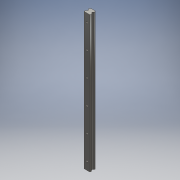
# Autodesk Inventor part: [Z] HGR15R
Saved by Autodesk Inventor 2016 (Build 200138000, 138)
## iProperties
Created: 2013-03-18
Part Number: [Z] HGR15R
Material: Сталь
Description: SolidWorks IGES file using analytic representation for surfaces
Document SubType Name: Modeling
Designer: stan
Density: 7.85 g/cm^3
Appearance: Сталь — полированная
Sending System: SolidWorks 2012
Preprocessor: SolidWorks 2012
Minimum Resolution: 0.0
Sending System Product ID: HGR15R.SLDPRT
Receiving System Product ID: HGR15R.SLDPRT
Sent Units: Millimeter
Translation Standard: IGES 5.3
Model Creation Time: 2013-03-18
Autodesk Inventor part; units mm, degrees
ref_plane "YZ Plane" through (0, 0, 0) normal (1, 0, 0) x (0, 1, 0)
ref_plane "XZ Plane" through (0, 0, 0) normal (0, 1, 0) x (-1, 0, 0)
ref_plane "XY Plane" through (0, 0, 0) normal (0, 0, 1) x (1, 0, 0)
ref_plane "РабПлоскость1" through (-6.8, -15, 75) normal (0, 0, 1) x (1, 0, 0)
sketch "Эскиз2" plane through (-6.8, -15, 75) normal (0, 0, 1) x (1, 0, 0)
  arc A0 (11.9032, 8.6142) -> (12.017, 8.8451) centre (11.6204, 8.897) ccw projected
  arc A1 (13.5419, 10.2529) -> (12.017, 8.8451) centre (13.6233, 8.6349) ccw projected
  line L0 (14.3, 11.011) -> (13.5419, 10.2529) projected
  line L1 (14.3, 12.549) -> (14.3, 11.011) projected
  line L2 (13.5304, 13.3186) -> (14.3, 12.549) projected
  arc A2 (12.0183, 14.7157) -> (13.5304, 13.3186) centre (13.6233, 14.936) ccw projected
  arc A3 (12.0183, 14.7157) -> (11.9049, 14.9441) centre (11.622, 14.6613) ccw projected
  line L3 (11.849, 15) -> (11.9049, 14.9441) projected
  line L4 (11.849, 15) -> (1.751, 15) projected
  line L5 (1.6951, 14.9441) -> (1.751, 15) projected
  arc A4 (1.6951, 14.9441) -> (1.5817, 14.7157) centre (1.978, 14.6613) ccw projected
  arc A5 (0.0696, 13.3186) -> (1.5817, 14.7157) centre (-0.0233, 14.936) ccw projected
  line L6 (-0.7, 12.549) -> (0.0696, 13.3186) projected
  line L7 (-0.7, 11.011) -> (-0.7, 12.549) projected
  line L8 (0.0581, 10.2529) -> (-0.7, 11.011) projected
  arc A6 (1.583, 8.8451) -> (0.0581, 10.2529) centre (-0.0233, 8.6349) ccw projected
  arc A7 (1.583, 8.8451) -> (1.6968, 8.6142) centre (1.9796, 8.897) ccw projected
  line L9 (1.9128, 8.3982) -> (1.6968, 8.6142) projected
  arc A8 (2.03, 8.1153) -> (1.9128, 8.3982) centre (1.63, 8.1153) ccw projected
  line L10 (2.03, 6.5533) -> (2.03, 8.1153) projected
  arc A9 (1.9128, 6.2704) -> (2.03, 6.5533) centre (1.63, 6.5533) ccw projected
  line L11 (1.9128, 6.2704) -> (-0.4071, 3.9505) projected
  arc A10 (-0.4071, 3.9505) -> (-0.7, 3.2434) centre (0.3, 3.2434) ccw projected
  line L12 (-0.7, 3.2434) -> (-0.7, 0.7) projected
  line L13 (-0.7, 0.7) -> (0, 0) projected
  line L14 (13.6, 0) -> (0, 0) projected
  line L15 (13.6, 0) -> (14.3, 0.7) projected
  line L16 (14.3, 0.7) -> (14.3, 3.2434) projected
  arc A11 (14.3, 3.2434) -> (14.0071, 3.9505) centre (13.3, 3.2434) ccw projected
  line L17 (14.0071, 3.9505) -> (11.6872, 6.2704) projected
  arc A12 (11.57, 6.5533) -> (11.6872, 6.2704) centre (11.97, 6.5533) ccw projected
  line L18 (11.57, 8.1153) -> (11.57, 6.5533) projected
  arc A13 (11.6872, 8.3982) -> (11.57, 8.1153) centre (11.97, 8.1153) ccw projected
  line L19 (11.9032, 8.6142) -> (11.6872, 8.3982) projected
  point P0 (6.8, 15)
extrude "Выдавливание1" add sketch "Эскиз2" along normal blind 340
sketch "Эскиз3" plane through (-5.049, 0, 75) normal (0, 1, 0) x (1, 0, 0)
  line L0 (10.098, 0) -> (0, 0) projected
  line L1 (12.549, 0) -> (12.549, -340) projected
  point P0 (5.049, 75)
  point P1 (5.049, -20)
  point P2 (5.049, -80)
  point P3 (5.049, -140)
  point P4 (5.049, -200)
  point P5 (5.049, -260)
  point P6 (5.049, -320)
  dimension "d2" = 20
  dimension "d3" = 7.5
  dimension "d6" = 60
  constraints: 1 vertical, 5 other
  measures "d2" distance from line of point (5.049, -20) L0
  measures "d3" distance from line of point (5.049, -20) L1
  measures "d6" distance of point (5.049, -20) point (5.049, -80)
hole "Отверстие1" at (0, 0, 95) at (0, 0, 155) at (0, 0, 215) at (0, 0, 275) at (0, 0, 335) at (0, 0, 395) direction (0, -1, 0) diameter 4.5 end through all counterbore diameter 7.5 counterbore depth 5.3
